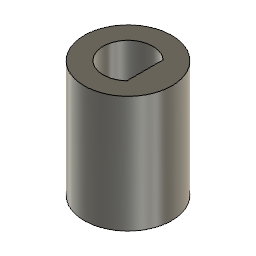
motor_coupler (Autodesk Fusion 360 design; units mm, degrees)
Autodesk Fusion 360 part; units mm, degrees
sketch "Sketch5" plane through (0, 0, 0) normal (0, 0, 1) x (1, 0, 0)
  circle A0 centre (0, 0) radius 7.5
  line L0 (1.7, 2.1616) -> (1.7, -2.1616)
  arc A1 (1.7, 2.1616) -> (1.7, -2.1616) centre (0, 0) ccw
  dimension "d19" = 15
  dimension "d29" = 5.5
  dimension "d30" = 1.7
  constraint coincident A0.centre A1.centre
  constraint vertical L0
  measures "d19" diameter of A0
  measures "d29" diameter of A1
  measures "d30" distance of A0.centre L0
extrude "Extrude7" add sketch "Sketch5" along normal blind 10
sketch "Sketch7" plane through (0, 0, 10) normal (0, 0, 1) x (-1, 0, 0)
  arc A0 (-1.7, -2.1616) -> (-1.7, 2.1616) centre (0, 0) ccw
  line L0 (-1.7, -2.1616) -> (-1.7, 2.1616)
  circle A1 centre (0, 0) radius 7.5
  circle A2 centre (0, 0) radius 7.5
  line L1 (-2.9, -3.1068) -> (-2.9, 3.1068)
  arc A3 (-2.9, -3.1068) -> (-2.9, 3.1068) centre (0, 0) ccw
  dimension "d35" = 8.5
  dimension "d36" = 2.9
  constraint coincident A0.centre A1.centre
  constraint vertical L1
  measures "d35" diameter of A3
  measures "d36" distance of A0.centre L1
extrude "Extrude8" add sketch "Sketch7" along normal blind 10 contours A1 A2
